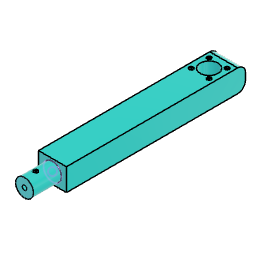
Braço robótico 3.0(cerra) v15 (Autodesk Fusion 360 design; units mm, degrees)
Autodesk Fusion 360 part; units mm, degrees
sketch "Sketch4" plane through (0, 0, 0) normal (0, 0, 1) x (1, 0, 0)
  line L0 (-200, 100) -> (-175, 100)
  line L1 (-175, 100) -> (-175, -60)
  line L2 (-175, -60) -> (-200, -60)
  line L3 (-200, -60) -> (-200, 100)
  dimension "d3" = 25
  dimension "d4" = 160
  constraint horizontal L0
  constraint vertical L1
  constraint horizontal L2
  constraint vertical L3
  measures "d3" distance of L0.start L0.end
  measures "d4" distance of L0.start L2.end
extrude "Extrude1" add sketch "Sketch4" along normal blind 20
sketch "Sketch5" plane through (0, 0, 20) normal (0, 0, 1) x (-1, 0, 0)
  line L0 (200, 60) -> (175, 60)
  line L1 (175, 60) -> (175, -100)
  line L2 (175, -100) -> (200, -100)
  line L3 (200, -100) -> (200, 60)
  circle A0 centre (187.5, -80) radius 8.0085
  dimension "d8" = 16.017
  measures "d8" diameter of A0
extrude "Extrude2" cut sketch "Sketch5" against normal blind 55 contours A0
fillet "Fillet1" radius 7 2 edges at (-187.5, 100, 20) (-187.5, 100, 0)
sketch "Sketch11" plane through (0, 0, 20) normal (0, 0, 1) x (-1, 0, 0)
  line L0 (200, -93) -> (200, 60)
  line L1 (200, 60) -> (175, 60)
  line L2 (175, 60) -> (175, -93)
  circle A0 centre (187.5, -80) radius 8.0085
  line L3 (187.5, -80) -> (179.4991, -88.0009)
  line L4 (187.5, -80) -> (195.5009, -88.0009)
  line L5 (187.5, -80) -> (195.5009, -71.9991)
  line L6 (187.5, -80) -> (179.4991, -71.9991)
  line L7 (175, -93) -> (200, -93)
hole "Hole2" at (-179.4991, 71.9991, 20) at (-179.4991, 88.0009, 20) at (-195.5009, 88.0009, 20) at (-195.5009, 71.9991, 20) direction (0, 0, -1) diameter 1.623 depth 20 tip angle 180 counterbore diameter 3.9 counterbore depth 1
thread "Thread3" "ISO Metric profile 2.0 M2x0.4 6H"
sketch "Sketch13" plane through (0, -60, 0) normal (0, -1, 0) x (1, 0, 0)
  line L0 (-200, 0) -> (-175, 0)
  line L1 (-175, 0) -> (-175, 20)
  line L2 (-175, 20) -> (-200, 20)
  line L3 (-200, 20) -> (-200, 0)
  circle A0 centre (-187.5, 10) radius 8
  dimension "d46" = 16
  measures "d46" diameter of A0
extrude "Extrude8" add sketch "Sketch13" along normal blind 25 contours A0
sketch "Sketch14" plane through (0, -85, 0) normal (0, -1, 0) x (1, 0, 0)
  circle A0 centre (-187.5, 10) radius 8
  circle A1 centre (-187.5, 10) radius 2.0005
  dimension "d49" = 4.001
  constraint concentric A0 A1
  measures "d49" diameter of A1
extrude "Extrude9" cut sketch "Sketch14" against normal blind 15 contours A1
sketch "Sketch16" plane through (0, -85, 0) normal (0, -1, 0) x (1, 0, 0)
  circle A0 centre (-187.5, 10) radius 2.0005
  circle A1 centre (-187.5, 10) radius 8
  circle A2 through (-179.5, 10, -25) (-191.5, 16.9282, -25) (-191.5, 3.0718, -25)
hole "Hole4" at (-187.5, -75.0094, 18) direction (0, 0, -1) diameter 1.623 end through all counterbore diameter 4 counterbore depth 1
thread "Thread5" "ISO Metric profile 2.0 M2x0.4 6H"
component "4124A15_7-1 4 Diameter Smooth-Cut Circular Saw Blade for Wood" placed x (1, 0, 0) y (0, 1, 0) z (0, 0, 1) at (0, 0, 0)
component "6343K96_Bearing Locknut" placed x (1, 0, 0) y (0, 0, -1) z (0, 1, 0) at (-164.7507, -187.0518, -22.2618)
component "6627T34_Stepper Motor" placed x (1, 0, 0) y (0, 1, 0) z (0, 0, 1) at (-161.9415, -183.813, -21.8716)
